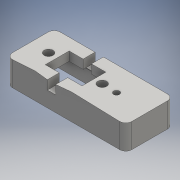
# Autodesk Inventor part: optical endstop top
Saved by Autodesk Inventor 2016 SP1 (Build 200210100, 210)
## iProperties
Created: 2016-04-16
Part Number: optical endstop top
Material: Generic
Document SubType Name: Modeling
Designer: ubik
Density: 1 g/cm^3
Appearance: Default
Author: ubik
Autodesk Inventor part; units mm, degrees
ref_plane "YZ Plane" through (0, 0, 0) normal (1, 0, 0) x (0, 1, 0)
ref_plane "XZ Plane" through (0, 0, 0) normal (0, 1, 0) x (-1, 0, 0)
ref_plane "XY Plane" through (0, 0, 0) normal (0, 0, 1) x (1, 0, 0)
ref_plane "Work Plane1" through (0, 0, 0) normal (0, 0, 1) x (1, 0, 0)
sketch "Sketch1" plane through (0, 0, 0) normal (0, 0, 1) x (1, 0, 0)
  circle A0 centre (-17.75, 4.5) radius 1.5 projected
  arc A1 (-25.75, 8) -> (-27.75, 6) centre (-25.75, 6) ccw projected
  line L0 (-27.75, 3) -> (-27.75, 6) projected
  line L1 (-30.85, 1) -> (-29.75, 1)
  arc A2 (-30.85, 1) -> (-32.85, -1) centre (-30.85, -1) ccw projected
  line L2 (-32.85, -13) -> (-32.85, -1) projected
  arc A3 (-32.85, -13) -> (-30.85, -15) centre (-30.85, -13) ccw projected
  line L3 (5.15, -15) -> (-30.85, -15) projected
  arc A4 (5.15, -15) -> (7.15, -13) centre (5.15, -13) ccw projected
  line L4 (7.15, -1) -> (7.15, -13) projected
  arc A5 (7.15, -1) -> (5.15, 1) centre (5.15, -1) ccw projected
  line L5 (-30.85, 1) -> (5.15, 1)
  line L6 (-7.75, 3) -> (-7.75, 6) projected
  arc A6 (-7.75, 6) -> (-9.75, 8) centre (-9.75, 6) ccw projected
  line L7 (-25.75, 8) -> (-9.75, 8) projected
  circle A7 centre (-8.75, -7) radius 1.5 projected
  circle A8 centre (-26.75, -7) radius 1.5 projected
  line L8 (-30.85, -12) -> (-5.5342, -12)
  line L9 (-30.85, -2) -> (-30.85, -12)
  line L10 (-5.5342, -2) -> (-5.5342, -12)
  line L11 (-5.5342, -2) -> (-30.85, -2)
  line L12 (-11.5342, -2) -> (-11.5342, -12)
  line L13 (-23.85, -2) -> (-23.85, -12)
  point P0 (0, 0)
  dimension "d2" = 6
  dimension "d3" = 12.6842
  dimension "d4" = 2
  dimension "d5" = 7
  constraints: 16 end point, 4 point on line, 2 perpendicular, 1 point on circle, 1 vertical
  measures "d2" distance between parallel lines of L12 L10
  measures "d3" distance between parallel lines of L10 L4
  measures "d4" distance between parallel lines of L2 L9
  measures "d5" distance between parallel lines of L9 L13
extrude "Extrusion4" add sketch "Sketch1" along normal blind 5.2 contours L1 L5 A5 L4 A4 L3 A3 L2 A2
sketch "Sketch5" plane through (0, 0, 5.2) normal (0, 0, 1) x (1, 0, 0)
  line L0 (-30.85, -3) -> (-23.85, -3)
  line L1 (-5.5342, -3) -> (-5.5342, -11)
  line L2 (-5.5342, -11) -> (-11.5342, -11)
  line L3 (-30.85, -11) -> (-30.85, -3)
  arc A0 (-30.85, 1) -> (-32.85, -1) centre (-30.85, -1) ccw projected
  line L4 (-32.85, -1) -> (-32.85, -13) projected
  arc A1 (-32.85, -13) -> (-30.85, -15) centre (-30.85, -13) ccw projected
  line L5 (-30.85, -15) -> (5.15, -15) projected
  arc A2 (5.15, -15) -> (7.15, -13) centre (5.15, -13) ccw projected
  line L6 (7.15, -13) -> (7.15, -1) projected
  arc A3 (7.15, -1) -> (5.15, 1) centre (5.15, -1) ccw projected
  line L7 (5.15, 1) -> (-30.85, 1) projected
  line L8 (-11.5342, -15) -> (-11.5342, 1)
  line L9 (-23.85, -15) -> (-23.85, 1)
  circle A4 centre (-8.75, -7) radius 1.5 projected
  circle A5 centre (-26.75, -7) radius 1.5 projected
  line L10 (-11.5342, -3) -> (-5.5342, -3)
  line L11 (-23.85, -3) -> (-11.5342, -3)
  line L12 (-11.5342, -11) -> (-23.85, -11)
  line L13 (-23.85, -11) -> (-30.85, -11)
  point P0 (0, 0)
  point P1 (-11.5342, -14)
  point P2 (-11.5342, 2)
  point P3 (-23.85, -14)
  point P4 (-23.85, 2)
  dimension "d16" = 6
  dimension "d17" = 7
  dimension "d22" = 4
  dimension "d23" = 4
  constraints: 20 end point, 6 point on line, 4 centre point, 6 other
  measures "d16" distance between parallel lines of L8 L1
  measures "d17" distance between parallel lines of L3 L9
extrude "Extrusion5" add sketch "Sketch5" along normal blind 3 contours L3 L13 L9 L5 A1 L4 A0 L7 L0 | L0 L9 L13 L3 | L9 L7 L8 L11 | L12 L8 L5 L9 | L10 L1 L2 L8 | L8 L7 A3 L6 A2 L5 L2 L1 L10
sketch "Sketch6" plane through (0, 0, 8.2) normal (0, 0, 1) x (1, 0, 0)
  line L0 (-16.35, -15) -> (-16.35, 1)
  line L1 (-19.15, -15) -> (-19.15, 1)
  line L2 (5.15, 1) -> (-30.85, 1)
  line L3 (-30.85, -15) -> (5.15, -15)
  point P0 (0, 0)
  constraints: 8 end point, 4 point on line
extrude "Extrusion6" cut sketch "Sketch6" against normal blind 3
sketch "Sketch7" plane through (0, 0, 0) normal (0, 0, -1) x (-1, 0, 0)
  line L0 (5.5342, -2) -> (30.85, -2) projected
  line L1 (30.85, -2) -> (30.85, -12) projected
  line L2 (30.85, -12) -> (5.5342, -12) projected
  line L3 (5.5342, -12) -> (5.5342, -2) projected
  line L4 (4.5342, -12.5) -> (31.35, -12.5)
  line L5 (31.35, -12.5) -> (31.35, -1.5)
  line L6 (31.35, -1.5) -> (4.5342, -1.5)
  line L7 (4.5342, -1.5) -> (4.5342, -12.5)
  line L8 (4.5342, -12.5) -> (-5.2525, -12.5)
  line L9 (-5.2525, -12.5) -> (-5.2525, -1.5)
  line L10 (-5.2525, -1.5) -> (4.5342, -1.5)
  line L11 (4.5342, -1.5) -> (4.5342, -12.5)
  point P0 (0, 0)
  dimension "d24" = 0.5
  dimension "d31" = 1
  constraints: 16 end point, 2 parallel, 1 horizontal, 1 perpendicular, 2 other
  measures "d24" distance between parallel lines of L2 L4
  measures "d31" distance between parallel lines of L7 L3
extrude "Extrusion7" cut sketch "Sketch7" against normal blind 5
sketch "Sketch8" plane through (0, 0, 8.2) normal (0, 0, 1) x (1, 0, 0)
  circle A0 centre (-3.75, -7.199) radius 1
  circle A1 centre (-8.75, -7) radius 1.5 projected
  point P0 (0, 0)
  dimension "d27" = 2
  dimension "d28" = 5
  constraints: 1 centre point
  measures "d27" diameter of A0
  measures "d28" horizontal distance of A1.centre A0.centre
extrude "Extrusion8" cut sketch "Sketch8" against normal through all contours A0
body "Solid1"
